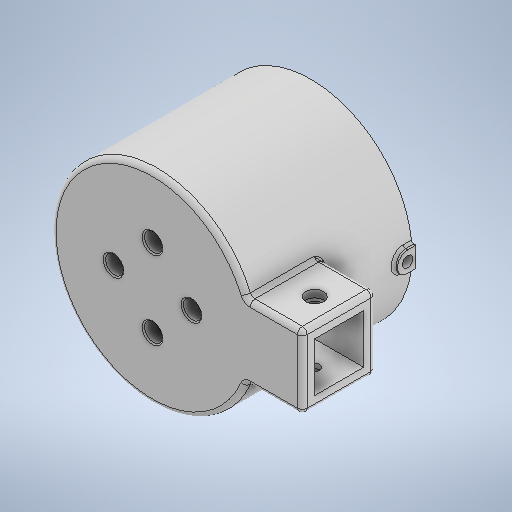
# Autodesk Inventor part: j3 moving part 2 option
Saved by Autodesk Inventor 2025 (Build 290162000, 162)
## iProperties
Created: 2025-07-29
Part Number: j3 moving part 2 option
Material: 一般
Document SubType Name: Modeling
Designer: gavin
Density: 1 g/cm^3
Appearance: 預設
Author: gavin
## iProperties of the stored document j3 moving part_3D 列印.ipt
Created: 2025-08-04
Part Number: j3 moving part_3D 列印
Material: 一般
Document SubType Name: Modeling
Designer: gavin
Density: 1 g/cm^3
Appearance: 預設
Author: gavin
Autodesk Inventor part; units mm, degrees
ref_plane "YZ Plane" through (0, 0, 0) normal (1, 0, 0) x (0, 1, 0)
ref_plane "XZ Plane" through (0, 0, 0) normal (0, 1, 0) x (-1, 0, 0)
ref_plane "XY Plane" through (0, 0, 0) normal (0, 0, 1) x (1, 0, 0)
sketch "草圖1" plane through (0, 0, 0) normal (0, 0, 1) x (1, 0, 0)
  circle A0 centre (0, 0) radius 37.575
  circle A1 centre (0, 0) radius 41.575
  dimension "d0" = 75.15
  dimension "d1" = 83.15
  constraints: 2 centre point, 2 coincident
  measures "d0" diameter of A0
  measures "d1" diameter of A1
extrude "擠出1" add sketch "草圖1" along normal blind 16
sketch "草圖2" plane through (0, 0, 16) normal (0, 0, 1) x (1, 0, 0)
  circle A0 centre (0, 0) radius 41.575 projected
  circle A1 centre (0, 0) radius 37.575 projected
  circle A2 centre (0, 0) radius 33.075
  dimension "d4" = 66.15
  constraints: 1 centre point, 1 coincident
  measures "d4" diameter of A2
extrude "擠出2" add sketch "草圖2" along normal blind 28.5 contours A0 | A1
sketch "草圖4" plane through (0, 0, 44.5) normal (0, 0, 1) x (1, 0, 0)
  circle A0 centre (0, 0) radius 41.575 projected
extrude "擠出3" add sketch "草圖4" along normal blind 15
sketch "草圖5" plane through (0, 0, 59.5) normal (0, 0, 1) x (1, 0, 0)
  circle A0 centre (0, 0) radius 41.575 projected
extrude "擠出4" add sketch "草圖5" along normal blind 5.575
sketch "草圖6" plane through (0, 0, 65.075) normal (0, 0, 1) x (1, 0, 0)
  circle A0 centre (0, 0) radius 41.575 projected
  line L0 (61.575, -15.075) -> (61.575, 15.075)
  line L1 (61.575, 15.075) -> (38.7456, 15.075)
  line L2 (61.575, -15.075) -> (38.7456, -15.075)
  point P0 (41.575, 0)
  point P1 (61.575, 0)
  dimension "d11" = 20
  dimension "d12" = 30.15
  constraints: 6 end point, 3 point on circle, 1 horizontal, 1 horizontal alignment, 1 midpoint, 1 perpendicular, 1 vertical
  measures "d11" distance of point (61.575, 0) A0.start
  measures "d12" distance of L0.start L0.end
extrude "擠出5" add sketch "草圖6" against normal blind 30.15 contours A0 L1 L0 L2
sketch "草圖7" plane through (0, 0, 65.075) normal (0, 0, 1) x (1, 0, 0)
  circle A0 centre (0, 0) radius 16 construction
  circle A1 centre (0, 16) radius 2.1
  circle A2 centre (-16, 0) radius 2.1
  circle A3 centre (0, -16) radius 2.1
  circle A4 centre (16, 0) radius 2.1
  dimension "d15" = 32
  dimension "d16" = 4.2
  dimension "d19" = 360
  constraints: 4 centre point, 1 coincident, 1 vertical alignment, 11 other
  measures "d16" diameter of A1
extrude "擠出6" cut sketch "草圖7" against normal through all
sketch "草圖8" plane through (0, 0, 65.075) normal (0, 0, 1) x (1, 0, 0)
  circle A0 centre (0, 16) radius 2.1 projected
  circle A1 centre (0, 16) radius 3.75
  circle A2 centre (-16, 0) radius 3.75
  circle A3 centre (0, -16) radius 3.75
  circle A4 centre (16, 0) radius 3.75
  point P0 (0, 0)
  dimension "d23" = 7.5
  dimension "d26" = 360
  constraints: 4 centre point, 1 coincident, 9 other
  measures "d23" diameter of A1
extrude "擠出7" cut sketch "草圖8" against normal blind 13.5 contours A0 | A1 | A2 | A3 | A4
chamfer "倒角1" distance 0.5 angle 45 4 edges at (-3.75, 16, 65.075) (-19.75, 0, 65.075) (12.25, 0, 65.075) (-3.75, -16, 65.075)
sketch "草圖9" plane through (61.575, -15.075, 65.075) normal (1, 0, 0) x (0, 0, -1)
  line L0 (0, 0) -> (0, 30.15) projected
  line L1 (0, 0) -> (30.15, 0) projected
  line L2 (30.15, 30.15) -> (30.15, 0) projected
  line L3 (0, 30.15) -> (30.15, 30.15) projected
  line L4 (25.15, 25.15) -> (25.15, 5)
  line L5 (25.15, 5) -> (5, 5)
  line L6 (5, 5) -> (5, 25.15)
  line L7 (5, 25.15) -> (25.15, 25.15)
  point P0 (65.075, 15.075)
  dimension "d33" = 5
  constraints: 8 end point, 3 other
  measures "d33" distance between parallel lines of L3 L7
extrude "擠出8" cut sketch "草圖9" against normal blind 20 contours L4 L5 L6 L7
fillet "圓角1" radius 2 9 edges at (-41.575, 0, 65.075) (50.1603, 15.075, 65.075) (61.575, 0, 65.075) (50.1603, -15.075, 65.075) (61.575, 15.075, 50) (61.575, 0, 34.925) (61.575, -15.075, 50) (38.7456, 15.075, 50) (38.7456, -15.075, 50)
sketch "草圖10" plane through (0, 0, 34.925) normal (0, 0, -1) x (-1, 0, 0)
  line L0 (-59.575, -15.075) -> (-59.575, 15.075) projected
  line L1 (-59.575, -15.075) -> (-40.0902, -15.075) projected
  arc A0 (-38.2502, -16.2913) -> (-40.0902, -15.075) centre (-40.0902, -17.075) ccw projected
  arc A1 (-38.2502, 16.2913) -> (-38.2502, -16.2913) centre (0, 0) ccw projected
  arc A2 (-40.0902, 15.075) -> (-38.2502, 16.2913) centre (-40.0902, 17.075) ccw projected
  line L2 (-40.0902, 15.075) -> (-59.575, 15.075) projected
  line L3 (-43.1398, 6) -> (-43.1398, -6)
  line L4 (-43.1398, -6) -> (-41.1398, -6)
  line L5 (-43.1398, 6) -> (-41.1398, 6)
  point P0 (-43.1398, 0)
  point P1 (-41.575, 0)
  dimension "d37" = 12
  dimension "d38" = 2
  constraints: 6 end point, 3 point on circle, 1 horizontal, 1 horizontal alignment, 1 midpoint, 1 perpendicular, 1 vertical
  measures "d37" distance of L3.start L3.end
  measures "d38" distance of L3.end L4.end
extrude "擠出9" add sketch "草圖10" along normal up to surface (34.925 mm away) contours L4 L3 L5 A1
sketch "草圖11" plane through (43.1398, -6, 34.925) normal (1, 0, 0) x (0, 0, -1)
  line L0 (34.925, 12) -> (34.925, 0) projected
  line L1 (0, 12) -> (34.925, 12) projected
  line L2 (0, 0) -> (0, 12) projected
  line L3 (0, 0) -> (34.925, 0) projected
  circle A0 centre (3.4625, 6) radius 2.165
  circle A1 centre (31.4625, 6) radius 2.165
  line L4 (3.4625, 6) -> (31.4625, 6)
  point P0 (34.925, 6)
  point P1 (17.4625, 6)
  point P2 (17.4625, 12)
  dimension "d41" = 4.33
  dimension "d42" = 4.33
  dimension "d43" = 28
  constraints: 2 centre point, 2 end point, 2 midpoint, 1 horizontal, 1 vertical alignment
  measures "d41" diameter of A0
  measures "d42" diameter of A1
  measures "d43" distance of L4.end L4.start
extrude "擠出10" cut sketch "草圖11" against normal blind 10 contours A0 | A1
fillet "圓角3" radius 2 6 edges at (38.9874, -15.4066, 34.925) (60.9892, -14.4892, 35.5108) (49.8326, -15.075, 34.925) (60.9892, 14.4892, 35.5108) (38.9874, 15.4066, 34.925) (49.8326, 15.075, 34.925)
sketch "草圖12" plane through (43.1398, -6, 34.925) normal (1, 0, 0) x (0, 0, -1)
  circle A0 centre (31.4625, 6) radius 2.165 projected
  circle A1 centre (3.4625, 6) radius 2.165 projected
  line L0 (34.925, 12) -> (34.925, 0) projected
  line L1 (0, 12) -> (34.925, 12) projected
  line L2 (0, 0) -> (0, 12) projected
  line L3 (0, 0) -> (34.925, 0) projected
  circle A2 centre (3.4625, 6) radius 4.165
  circle A3 centre (31.4625, 6) radius 4.165
  line L4 (0, -7.075) -> (0, 19.075) projected
  line L5 (3.4625, 10.165) -> (0, 10.165)
  line L6 (3.4625, 1.835) -> (0, 1.835)
  line L7 (31.4625, 10.165) -> (34.925, 10.165)
  line L8 (34.925, 12) -> (34.925, 0) projected
  line L9 (31.4625, 1.835) -> (34.925, 1.835)
  line L10 (34.925, 12) -> (34.925, 10.165)
  line L11 (34.925, 0) -> (0, 0) projected
  line L12 (34.925, 1.835) -> (34.925, 0)
  point P0 (34.925, 6)
  dimension "d48" = 2
  dimension "d49" = 2
  constraints: 12 end point, 8 point on line, 4 point on circle, 2 centre point, 2 collinear, 2 perpendicular, 1 tangent
  measures "d48" radial gap between concentric circles of A3 A0
  measures "d49" radial gap between concentric circles of A1 A2
extrude "擠出11" cut sketch "草圖12" against normal up to surface contours L0 L7 A3 L9 L3 L2 L6 A2 L5 L1 round surface about axis through (0, 0, 0) along (0, 0, 1) radius 41.575 far side no
fillet "圓角4" radius 1 14 edges at (38.7798, 14.9869, 35.6427) (40.6548, 8.6989, 34.925) (41.4536, -3.175, 28.7669) (41.4537, 3.1732, 28.7647) (41.3658, -4.165, 33.1937) (41.3658, 4.165, 33.1937) (42.2528, 4.165, 34.925) (38.7798, -14.9869, 35.6427) (40.6548, -8.6989, 34.925) (42.2528, -4.165, 34.925) (41.3658, -4.165, 1.7313) (41.3658, 4.165, 1.7313) (41.4537, -3.1732, 6.1603) (41.4536, 3.175, 6.1581)
sketch "草圖13" plane through (40.0902, 15.075, 63.075) normal (0, 1, 0) x (1, 0, 0)
  line L0 (21.4848, 3) -> (21.4848, 23.15) projected
  line L1 (21.4848, 3) -> (1.4848, 3) projected
  line L2 (1.4848, 3) -> (1.4848, 23.15) projected
  line L3 (21.4848, 23.15) -> (1.4848, 23.15) projected
  circle A0 centre (11.4848, 13.075) radius 2.1
  point P0 (-40.0902, 63.075)
  dimension "d53" = 4.2
  constraints: 1 centre point
  measures "d53" diameter of A0
extrude "擠出12" cut sketch "草圖13" against normal through all contours A0
sketch "草圖14" plane through (40.0902, 15.075, 63.075) normal (0, 1, 0) x (1, 0, 0)
  circle A0 centre (11.4848, 13.075) radius 2.1 projected
  line L0 (0, 26.15) -> (19.4848, 26.15) projected
  line L1 (0, 0) -> (0, 26.15) projected
  line L2 (19.4848, 0) -> (0, 0) projected
  line L3 (19.4848, 26.15) -> (19.4848, 0) projected
  circle A1 centre (11.4848, 13.075) radius 3.65
  point P0 (-40.0902, 63.075)
  dimension "d56" = 7.3
  constraints: 1 centre point, 1 coincident
  measures "d56" diameter of A1
extrude "擠出13" cut sketch "草圖14" against normal blind 3 contours A1
mirror "鏡射1" about plane through (0, 0, 0) normal (0, 1, 0) of "擠出13"
sketch "草圖15" plane through (0, 0, 44.5) normal (0, 0, -1) x (-1, 0, 0)
  circle A0 centre (0, 0) radius 19.6
  dimension "d59" = 39.2
  constraints: 1 centre point, 1 coincident
  measures "d59" diameter of A0
extrude "擠出14" cut sketch "草圖15" against normal blind 2
